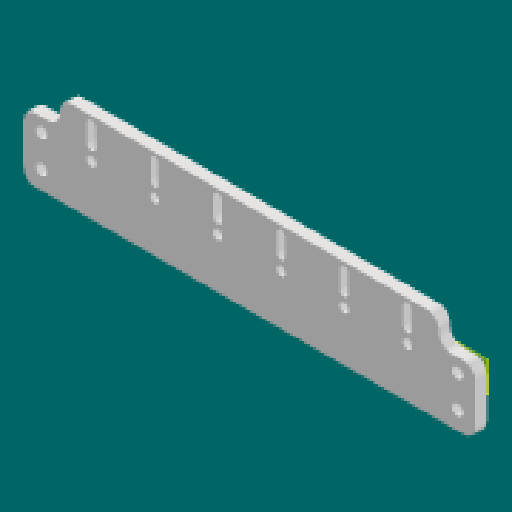
# Autodesk Inventor part: servo_mount_2
Saved by Autodesk Inventor 2023 (Build 270158000, 158)
## iProperties
Created: 2022-11-12
Part Number: servo_mount_2
Material: Generic
Document SubType Name: Modeling
Designer: sgodi
Density: 1 g/cm^3
Appearance: Default
Author: sgodi
Autodesk Inventor part; units mm, degrees
ref_plane "YZ Plane" through (0, 0, 0) normal (1, 0, 0) x (0, 1, 0)
ref_plane "XZ Plane" through (0, 0, 0) normal (0, 1, 0) x (-1, 0, 0)
ref_plane "XY Plane" through (0, 0, 0) normal (0, 0, 1) x (1, 0, 0)
ref_plane "Work Plane1" through (-42.5139, 0, 0) normal (0, 0, 1) x (1, 0, 0)
sketch "Sketch1" plane through (-42.5139, 0, 0) normal (0, 0, 1) x (1, 0, 0)
  line L0 (-61.9417, 0) -> (61.9417, 0)
  line L1 (61.9417, 0) -> (61.9417, -14.325)
  line L2 (58.7667, -17.5) -> (-58.7667, -17.5)
  line L3 (-61.9417, -14.325) -> (-61.9417, 0)
  line L4 (-61.9417, -14.325) -> (-61.9417, -7.5) projected
  line L5 (61.9417, -7.5) -> (61.9417, -14.325) projected
  line L6 (-75.2, -7.5) -> (75.2, -7.5) projected
  line L7 (-58.7667, 0) -> (-55.1167, 0) projected
  line L8 (55.1167, 0) -> (58.7667, 0) projected
  line L9 (-58.7667, -17.5) -> (-53.0564, -17.5) projected
  line L10 (53.0564, -17.5) -> (58.7667, -17.5) projected
  arc A0 (-61.9417, -14.325) -> (-58.7667, -17.5) centre (-58.7667, -14.325) ccw
  arc A1 (58.7667, -17.5) -> (61.9417, -14.325) centre (58.7667, -14.325) ccw
  circle A2 centre (-56.9417, -3.75) radius 1.524 projected
  circle A3 centre (-56.9417, -12.5) radius 1.524 projected
  circle A4 centre (56.9417, -12.5) radius 1.524 projected
  circle A5 centre (56.9417, -3.75) radius 1.524 projected
  line L11 (-43.3353, -7.5) -> (43.3353, -7.5)
  line L12 (43.3353, -7.5) -> (43.3353, -17.5)
  line L13 (43.3353, -17.5) -> (-43.3353, -17.5)
  line L14 (-43.3353, -17.5) -> (-43.3353, -7.5)
  line L15 (-43.3353, -11.5) -> (43.3353, -11.5) projected
  line L16 (-58.7667, -17.5) -> (-53.0564, -17.5) projected
  line L17 (-58.7667, -17.5) -> (-53.0564, -17.5) projected
  line L18 (53.0564, -17.5) -> (58.7667, -17.5) projected
  line L19 (43.3353, -7.5) -> (53.0564, -17.5)
  line L20 (-53.0564, -17.5) -> (-43.3353, -7.5)
  line L21 (-56.9417, -3.75) -> (56.9417, -3.75) construction
  line L22 (-51.9417, -7.5) -> (-51.9417, -3.175) projected
  line L23 (51.9417, -3.175) -> (51.9417, -7.5) projected
  circle A6 centre (-43.2848, -3.75) radius 1.27
  circle A7 centre (-25.9709, -3.75) radius 1.27
  circle A8 centre (-8.657, -3.75) radius 1.27
  circle A9 centre (8.657, -3.75) radius 1.27
  circle A10 centre (25.9709, -3.75) radius 1.27
  circle A11 centre (43.2848, -3.75) radius 1.27
  line L24 (-51.9417, 0) -> (51.9417, 0)
  line L25 (51.9417, 0) -> (51.9417, 7.112)
  line L26 (51.9417, 7.112) -> (-51.9417, 7.112)
  line L27 (-51.9417, 7.112) -> (-51.9417, 0)
  circle A12 centre (-43.2848, 0) radius 1.133
  circle A13 centre (-43.2848, 5) radius 1.133
  line L28 (-44.4178, 5) -> (-44.4178, 0)
  line L29 (-42.1518, 0) -> (-42.1518, 5)
  circle A14 centre (-25.9709, 0) radius 1.133
  circle A15 centre (-25.9709, 5) radius 1.133
  line L30 (-27.1039, 5) -> (-27.1039, 0)
  line L31 (-24.8379, 0) -> (-24.8379, 5)
  circle A16 centre (-8.657, 0) radius 1.133
  circle A17 centre (-8.657, 5) radius 1.133
  line L32 (-9.79, 5) -> (-9.79, 0)
  line L33 (-7.524, 0) -> (-7.524, 5)
  circle A18 centre (8.657, 0) radius 1.133
  circle A19 centre (8.657, 5) radius 1.133
  line L34 (7.524, 5) -> (7.524, 0)
  line L35 (9.79, 0) -> (9.79, 5)
  circle A20 centre (25.9709, 0) radius 1.133
  circle A21 centre (25.9709, 5) radius 1.133
  line L36 (24.8379, 5) -> (24.8379, 0)
  line L37 (27.1039, 0) -> (27.1039, 5)
  circle A22 centre (43.2848, 0) radius 1.133
  circle A23 centre (43.2848, 5) radius 1.133
  line L38 (42.1518, 5) -> (42.1518, 0)
  line L39 (44.4178, 0) -> (44.4178, 5)
  point P0 (42.5139, 0)
  point P1 (0, -3.75)
  point P2 (-27.1039, 0)
  point P3 (7.524, 0)
  point P4 (24.8379, 0)
  point P5 (27.1039, 0)
  point P6 (42.1518, 0)
  point P7 (44.4178, 0)
  point P8 (27.1039, 0)
  point P9 (24.8379, 0)
  point P10 (9.79, 0)
  point P11 (7.524, 0)
  point P12 (-7.524, 0)
  point P13 (-9.79, 0)
  point P14 (-24.8379, 0)
  point P15 (-27.1039, 0)
  point P16 (-42.1518, 0)
  dimension "d1" = 3.175
  dimension "d2" = 3.75
  dimension "d5" = 2.54
  dimension "d6" = 103.8834
  dimension "d10" = 17.3139
  dimension "d15" = 8.657
  dimension "d19" = 86.5695
  dimension "d20" = 8.657
  dimension "d21" = 7.112
  dimension "d22" = 2.266
  dimension "d23" = 2.266
  dimension "d25" = 5
  dimension "d29" = 17.3139
  constraints: 52 end point, 28 point on circle, 20 centre point, 8 tangent, 7 horizontal, 5 collinear, 5 parallel, 5 point on line, 2 perpendicular, 2 vertical alignment, 1 equal radius, 1 midpoint, 1 vertical, 65 other
  measures "d1" radius of A0
  measures "d2" distance from line of L6 L21.start
  measures "d5" diameter of A6
  measures "d6" distance between parallel lines of L23 L22
  measures "d10" distance of A6.centre A7.centre
  measures "d15" distance from line of L23 A11.centre
  measures "d19" distance of A11.centre A6.centre
  measures "d20" distance from line of L22 A6.centre
  measures "d21" distance of L24.end L25.end
  measures "d22" diameter of A12
  measures "d23" diameter of A13
  measures "d25" distance of A13.centre A12.centre
  measures "d29" distance of A12.centre A14.centre
extrude "Extrusion1" add sketch "Sketch1" along normal blind 3.175 contours L0 A12 A14 A16 A18 A20 A22 L1 L6 L3 | L6 L20 L2 A0 L3 | L27 L26 L25 L0 L39 A23 L38 L37 A21 L36 L35 A19 L34 L33 A17 L32 L31 A15 L30 L29 A13 L28 | L6 L12 L15 L14 | L14 L2 L20 | L19 L2 L12 | L6 L1 A1 L2 L19 | L15 L12 L2 L14
fillet "Fillet1" radius 3.175 6 edges at (9.4278, 0, 1.5875) (9.4278, 7.112, 1.5875) (-94.4556, 7.112, 1.5875) (-94.4556, 0, 1.5875) (-104.4556, 0, 1.5875) (19.4278, 0, 1.5875)
equation "\"d10\" = 0.166667 * d6"
equation "\"d20\" = -0.5 * d19 + 0.5 * d6"
equation "\"d23\" = d22"
equation "\"d29\" = d10"
body "Solid1"
